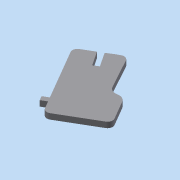
# Autodesk Inventor part: adelante
Saved by Autodesk Inventor 2015 (Build 190159000, 159)
## iProperties
Created: 2017-10-04
Part Number: adelante
Material: Generic
Document SubType Name: Modeling
Designer: Max
Density: 1 g/cm^3
Appearance: Default
Author: Max
Autodesk Inventor part; units mm, degrees
ref_plane "YZ Plane" through (0, 0, 0) normal (1, 0, 0) x (0, 1, 0)
ref_plane "XZ Plane" through (0, 0, 0) normal (0, 1, 0) x (-1, 0, 0)
ref_plane "XY Plane" through (0, 0, 0) normal (0, 0, 1) x (1, 0, 0)
sketch "Sketch1" plane through (0, 0, 0) normal (0, 0, 1) x (1, 0, 0)
  line L0 (-9.0847, 275.4971) -> (0.0597, 261.7096)
  line L1 (0.0597, 261.7096) -> (-4.5238, 258.6697)
  line L2 (-4.5238, 258.6697) -> (-13.846, 272.7251)
  line L3 (-20.4878, 268.8466) -> (-13.846, 272.7251)
  line L4 (-9.0847, 275.4971) -> (-3.3614, 279.1755)
  line L5 (-20.4878, 268.8466) -> (-29.1232, 263.8039)
  line L6 (-3.3614, 279.1755) -> (5.4134, 283.9717)
  line L7 (11.2184, 194.7202) -> (22.61, 201.3724)
  line L8 (44.4638, 214.134) -> (54.3957, 219.9338)
  line L9 (4.4881, 206.2457) -> (-0.6932, 203.2201)
  line L10 (-0.6932, 203.2201) -> (-3.2145, 207.5378)
  line L11 (-3.2145, 207.5378) -> (1.9667, 210.5634)
  line L12 (-29.1232, 263.8039) -> (1.9667, 210.5634)
  line L13 (4.4881, 206.2457) -> (11.2184, 194.7202)
  line L14 (54.3957, 219.9338) -> (37.2403, 249.3118)
  line L15 (37.2403, 249.3118) -> (27.3211, 243.8901)
  line L16 (27.3211, 243.8901) -> (5.4134, 283.9717)
  line L17 (44.4638, 214.134) -> (22.61, 201.3724)
  point P0 (0, 0)
  dimension "d11" = 20
  dimension "d12" = 5.5
  dimension "d13" = 10
  dimension "d14" = 80
  dimension "d15" = 50
  dimension "d16" = 10
  dimension "d17" = 6
  dimension "d18" = 5
  constraints: 36 end point, 8 perpendicular
  measures "d11" distance of L5.start L4.end
  measures "d12" distance between parallel lines of L0 L2
  measures "d13" distance of L5.start L12.start
  measures "d14" distance of L12.start L13.end
  measures "d15" distance of L13.end L14.start
  measures "d16" distance of L4.end L16.end
  measures "d17" distance of L9.start L9.end
  measures "d18" distance of L9.end L11.start
extrude "Extrusion1" add sketch "Sketch1" along normal blind 5.5
fillet "Fillet2" radius 8 2 edges at (37.2403, 249.3118, 2.75) (27.3211, 243.8901, 2.75)
fillet "Fillet3" radius 5 4 edges at (5.4134, 283.9717, 2.75) (54.3957, 219.9338, 2.75) (11.2184, 194.7202, 2.75) (-29.1232, 263.8039, 2.75)
body "Solid1"
